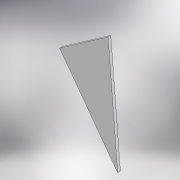
# Autodesk Inventor part: 2
Saved by Autodesk Inventor 2020 (Build 240168000, 168)
## iProperties
Created: 2019-05-26
Part Number: 2
Material: Generic
Document SubType Name: Modeling
Designer: chitl
Density: 1 g/cm^3
Appearance: Default
Author: chitl
Autodesk Inventor part; units mm, degrees
ref_plane "YZ Plane" through (0, 0, 0) normal (1, 0, 0) x (0, 1, 0)
ref_plane "XZ Plane" through (0, 0, 0) normal (0, 1, 0) x (-1, 0, 0)
ref_plane "XY Plane" through (0, 0, 0) normal (0, 0, 1) x (1, 0, 0)
sketch "Sketch1" plane through (0, 0, 0) normal (0, 0, 1) x (1, 0, 0)
  line L0 (-85.3293, 117.4307) -> (-13.5059, 167.8881)
  line L1 (-13.5059, 167.8881) -> (0.6992, 0.5848)
  line L2 (0.6992, 0.5848) -> (-85.3293, 117.4307)
  line L3 (-123.08, 47.6293) -> (-85.3293, 117.4307)
  line L4 (-123.4672, 47.5555) -> (0.6992, 0.5848)
  point P0 (0, 0)
  point P1 (0.6992, 0.5848)
  point P2 (-13.5059, 167.8881)
  constraints: 10 end point
extrude "Extrusion1" add sketch "Sketch1" along normal blind 4
body "Solid1"
